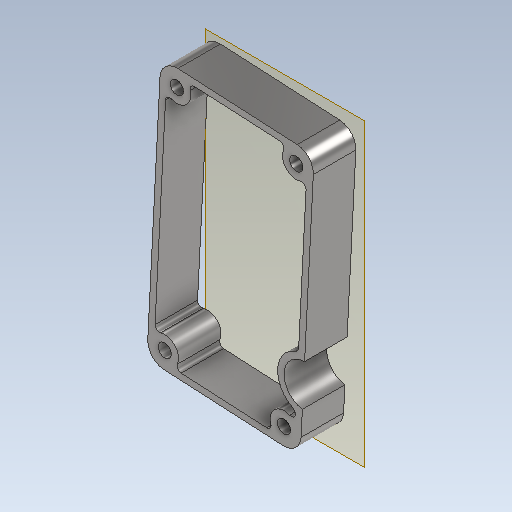
# Autodesk Inventor part: Стойка
Saved by Autodesk Inventor 2021 (Build 250183000, 183)
## iProperties
Created: 2020-12-07
Part Number: Стойка
Material: Сталь нержавеющая, 440C
Document SubType Name: Modeling
Designer: User
Density: 7.75 g/cm^3
Appearance: С умеренной полировкой
Author: User
Autodesk Inventor part; units mm, degrees
ref_plane "YZ Plane" through (0, 0, 0) normal (1, 0, 0) x (0, 1, 0)
ref_plane "XZ Plane" through (0, 0, 0) normal (0, 1, 0) x (-1, 0, 0)
ref_plane "РабПлоскость1" through (0, 0, 0) normal (0, 0, 1) x (1, 0, 0)
sketch "Эскиз1" plane through (0, 0, 0) normal (0, 0, 1) x (1, 0, 0)
  circle A0 centre (-30.9426, -53.5039) radius 3 construction
  circle A1 centre (25.1804, -56.4452) radius 3 construction
  circle A2 centre (-25.1804, 56.4452) radius 3 construction
  circle A3 centre (30.9426, 53.5039) radius 3 construction
  circle A4 centre (-30.9426, -53.5039) radius 3.1
  circle A5 centre (25.1804, -56.4452) radius 3.1
  circle A6 centre (30.9426, 53.5039) radius 3.1
  circle A7 centre (-25.1804, 56.4452) radius 3.1
  line L0 (38.9316, 53.0852) -> (34.8315, -25.15)
  arc A8 (38.9316, 53.0852) -> (31.3613, 61.493) centre (30.9426, 53.5039) ccw
  line L1 (-24.7617, 64.4342) -> (31.3613, 61.493)
  arc A9 (-24.7617, 64.4342) -> (-33.1694, 56.8639) centre (-25.1804, 56.4452) ccw
  line L2 (-38.9316, -53.0852) -> (-33.1694, 56.8639)
  arc A10 (-38.9316, -53.0852) -> (-31.3613, -61.493) centre (-30.9426, -53.5039) ccw
  line L3 (-8.2929, -62.7019) -> (-31.3613, -61.493)
  line L4 (24.7617, -64.4342) -> (11.6797, -63.7486)
  arc A11 (24.7617, -64.4342) -> (33.1694, -56.8639) centre (25.1804, -56.4452) ccw
  line L5 (33.7848, -45.1226) -> (33.1694, -56.8639)
  line L6 (11.6797, -63.7486) -> (-8.2929, -62.7019)
  arc A12 (34.8315, -25.15) -> (33.7848, -45.1226) centre (35.2069, -35.1834) ccw
  circle A13 centre (35.2069, -35.1834) radius 4 construction
  arc A14 (34.989, -22.1448) -> (33.6273, -48.1278) centre (35.2069, -35.1834) ccw
  line L7 (31.9635, -22.5528) -> (35.7184, 49.0946)
  circle A15 centre (30.9426, 53.5039) radius 6.5
  circle A16 centre (-25.1804, 56.4452) radius 6.5
  circle A17 centre (25.1804, -56.4452) radius 6.5
  circle A18 centre (-30.9426, -53.5039) radius 6.5
  line L8 (27.0566, 58.7144) -> (-20.7711, 61.221)
  line L9 (30.3909, -52.5593) -> (30.661, -47.4059)
  line L10 (20.7711, -61.221) -> (-27.0566, -58.7144)
  line L11 (-35.7184, -49.0946) -> (-30.3909, 52.5593)
  point P0 (0, 0)
  dimension "d2" = 6.2
  dimension "d6" = 6
  dimension "d9" = 6.2
  dimension "d10" = 6.2
  dimension "d11" = 6.2
  dimension "d12" = 10.0404
  dimension "d13" = 13.0404
  dimension "d14" = 3
  dimension "d15" = 13
  dimension "d16" = 3
  dimension "d17" = 3
  dimension "d18" = 3
  dimension "d19" = 3
  constraints: 24 end point, 22 point on circle, 15 centre point, 10 coincident, 5 parallel, 3 equal radius, 2 point on line, 28 other
  measures "d2" diameter of A4
  measures "d6" diameter of A0
  measures "d9" diameter of A5
  measures "d10" diameter of A6
  measures "d11" diameter of A7
  measures "d12" radius of A12
  measures "d13" radius of A14
  measures "d14" distance between parallel lines of L7 L0
  measures "d15" diameter of A15
  measures "d16" distance between parallel lines of L1 L8
  measures "d17" distance between parallel lines of L9 L5
  measures "d18" distance between parallel lines of L6 L10
  measures "d19" distance between parallel lines of L2 L11
ref_plane "РабПлоскость2" through (-53.0981, -74.1022, 20) normal (0, 0, -1) x (0.2079, 0.9781, 0)
extrude "Выдавливание1" add sketch "Эскиз1" along normal up to surface (20 mm away) contours L0 A14 L7 A15 L8 A16 L11 A18 L10 A17 L9 L5 A11 L4 L6 L3 A10 L2 A9 L1 A8 | L0 A12 L5 A14 | A15 | A17 | A16 | A18
fillet "Сопряжение1" radius 2 10 edges at (20.7711, -61.221, 10) (30.3909, -52.5593, 10) (-35.7184, -49.0946, 10) (-27.0566, -58.7144, 10) (27.0566, 58.7144, 10) (35.7184, 49.0946, 10) (-20.7711, 61.221, 10) (-30.3909, 52.5593, 10) (31.9635, -22.5528, 10) (30.661, -47.4059, 10)
equation "\"d9\" = d2"
equation "\"d10\" = d2"
equation "\"d11\" = d2"
